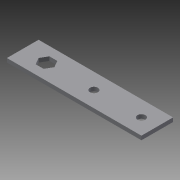
# Autodesk Inventor part: ArmBrace
Saved by Autodesk Inventor 2013 (Build 170138000, 138)
## iProperties
Created: 2014-01-29
Part Number: ArmBrace
Material: Generic
Document SubType Name: Modeling
Designer: 215152
Density: 1 g/cm^3
Author: 215152
Autodesk Inventor part; units mm, degrees
ref_plane "YZ Plane" through (0, 0, 0) normal (1, 0, 0) x (0, 1, 0)
ref_plane "XZ Plane" through (0, 0, 0) normal (0, 1, 0) x (-1, 0, 0)
ref_plane "XY Plane" through (0, 0, 0) normal (0, 0, 1) x (1, 0, 0)
sketch "Sketch1" plane through (0, 0, 0) normal (0, 1, 0) x (-1, 0, 0)
  line L0 (50.8, 12.7) -> (-50.8, 12.7)
  line L1 (-50.8, 12.7) -> (-50.8, -12.7)
  line L2 (-50.8, -12.7) -> (50.8, -12.7)
  line L3 (50.8, -12.7) -> (50.8, 12.7)
  line L4 (50.8, 12.7) -> (-50.8, -12.7) construction
  line L5 (-50.8, 12.7) -> (50.8, -12.7) construction
  point P0 (0, 0)
  dimension "d0" = 101.6
  dimension "d1" = 25.4
  constraints: 12 end point, 2 midpoint, 2 parallel, 1 horizontal, 1 perpendicular
  measures "d0" distance of L2.end L1.end
  measures "d1" distance of L1.end L0.end
extrude "Extrusion1" add sketch "Sketch1" along normal blind 3.175
sketch "Sketch2" plane through (0, 3.175, 0) normal (0, 1, 0) x (1, 0, 0)
  line L0 (-50.8, 12.7) -> (-50.8, -12.7) projected
  circle A0 centre (0, 0) radius 6.35
  line L1 (0, 0) -> (0, 6.35)
  line L2 (0, 0) -> (6.35, 0)
  line L3 (6.35, 0) -> (3.175, -5.4993)
  line L4 (3.175, -5.4993) -> (-3.175, -5.4993)
  line L5 (-3.175, -5.4993) -> (-6.35, 0)
  line L6 (-6.35, 0) -> (-3.175, 5.4993)
  line L7 (-3.175, 5.4993) -> (3.175, 5.4993)
  line L8 (3.175, 5.4993) -> (6.35, 0)
  dimension "d4" = 12.7
  constraints: 16 end point, 2 coincident, 2 point on circle, 1 centre point, 1 parallel, 1 perpendicular, 13 other
  measures "d4" diameter of A0
extrude "Extrusion2" cut sketch "Sketch2" against normal blind 3.175 contours L3 L4 L5 L6 L7 L1 L2 | L2 L1 L7 L8
sketch "Sketch3" plane through (0, 3.175, 0) normal (0, 1, 0) x (1, 0, 0)
  line L0 (50.8, 12.7) -> (-50.8, 12.7) projected
  line L1 (-50.8, 12.7) -> (-50.8, -12.7) projected
  line L2 (0, 0) -> (-38.1, 0)
  line L3 (-38.1, 0) -> (38.1, 0)
  circle A0 centre (-38.1, 0) radius 3.175
  circle A1 centre (38.1, 0) radius 3.175
  dimension "d7" = 38.1
  dimension "d8" = 76.2
  dimension "d9" = 0
  dimension "d10" = 6.35
  dimension "d11" = 6.35
  constraints: 4 end point, 2 centre point, 2 coincident, 1 parallel, 1 perpendicular
  measures "d7" distance of L2.start L2.end
  measures "d8" distance of L2.end L3.end
  measures "d9" distance between parallel lines of L3 L2
  measures "d10" diameter of A0
  measures "d11" diameter of A1
extrude "Extrusion3" cut sketch "Sketch3" against normal blind 3.175
sketch "Sketch4" plane through (0, 3.175, 0) normal (0, 1, 0) x (1, 0, 0)
  circle A0 centre (-38.1, 0) radius 3.175 projected
  line L0 (-50.8, 12.7) -> (-12.7, 12.7)
  line L1 (-12.7, 12.7) -> (-12.7, -12.7)
  line L2 (-12.7, -12.7) -> (-50.8, -12.7)
  line L3 (-50.8, -12.7) -> (-50.8, 12.7)
  point P0 (0, 0)
  dimension "d14" = 38.1
  dimension "d15" = 25.4
  constraints: 8 end point, 2 parallel, 1 horizontal, 1 perpendicular
  measures "d14" distance of L1.end L2.end
  measures "d15" distance of L0.end L1.end
extrude "Extrusion4" cut sketch "Sketch4" against normal blind 25.4
sketch "Sketch5" plane through (0, 3.175, 0) normal (0, 1, 0) x (1, 0, 0)
  circle A0 centre (38.1, 0) radius 3.175 projected
  line L0 (3.175, -5.4993) -> (-3.175, -5.4993) projected
  line L1 (38.1, 0) -> (76.2, 0)
  line L2 (38.1, 0) -> (76.2, 0) construction
  circle A1 centre (76.2, 0) radius 3.175
  line L3 (50.8, 12.7) -> (88.9, 12.7)
  line L4 (88.9, 12.7) -> (88.9, -12.7)
  line L5 (88.9, -12.7) -> (50.8, -12.7)
  line L6 (50.8, -12.7) -> (50.8, 12.7)
  point P0 (0, 0)
  dimension "d18" = 38.1
  dimension "d19" = 0
  dimension "d20" = 6.35
  dimension "d21" = 38.1
  dimension "d22" = 25.4
  constraints: 12 end point, 3 parallel, 2 horizontal, 1 centre point, 1 coincident, 1 collinear, 1 perpendicular
  measures "d18" distance of L1.start L1.end
  measures "d19" distance between parallel lines of L2 L1
  measures "d20" diameter of A1
  measures "d21" distance of L4.end L5.end
  measures "d22" distance of L3.end L4.end
extrude "Extrusion5" add sketch "Sketch5" against normal blind 3.175 contours L6 L3 L4 L5
sketch "Sketch6" plane through (-12.7, 3.175, -12.7) normal (-1, 0, 0) x (0, 0, 1)
  line L0 (25.4, -3.175) -> (0, -3.175) projected
  line L1 (25.4, 0) -> (25.4, -3.175) projected
  line L2 (0, 0) -> (25.4, 0) projected
  line L3 (0, -3.175) -> (0, 0) projected
  point P0 (12.7, -3.175)
extrude "Extrusion6" add sketch "Sketch6" along normal blind 6.35
body "Solid1"
